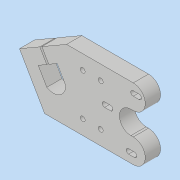
# Autodesk Inventor part: MMplate1
Saved by Autodesk Inventor 2017 (Build 210142000, 142)
## iProperties
Created: 2016-12-19
Part Number: MMplate1
Material: Generic
Document SubType Name: Modeling
Designer: Joshua Yuan
Density: 1 g/cm^3
Appearance: Default
Author: Joshua Yuan
Autodesk Inventor part; units mm, degrees
ref_plane "YZ Plane" through (0, 0, 0) normal (1, 0, 0) x (0, 1, 0)
ref_plane "XZ Plane" through (0, 0, 0) normal (0, 1, 0) x (-1, 0, 0)
ref_plane "XY Plane" through (0, 0, 0) normal (0, 0, 1) x (1, 0, 0)
sketch "sketch_plate" plane through (0, 0, 0) normal (0, 0, 1) x (1, 0, 0)
  line L0 (31.295, 48.2296) -> (38.3479, 52.3016)
  line L1 (47.1013, 57.4282) -> (54.2133, 45.1098)
  line L2 (31.295, 48.2296) -> (38.407, 35.9113)
  arc A0 (38.407, 35.9113) -> (54.2133, 45.1098) centre (43.8034, 44.8181) ccw
  line L3 (15.6813, 52.4133) -> (32.6329, 62.2003)
  line L4 (15.6813, 52.4133) -> (36.6325, 16.1248)
  line L5 (-9.4061, 0) -> (166.2056, 0) projected
  line L6 (0, -0.1502) -> (0, 91.4329) projected
  line L7 (34.3334, 63.2549) -> (40.0484, 53.3562)
  line L8 (32.6329, 62.2003) -> (38.3479, 52.3016)
  line L9 (34.3334, 63.2549) -> (54.8928, 75.1248)
  line L10 (40.0484, 53.3562) -> (47.1013, 57.4282)
  arc A1 (113.2079, 16.5197) -> (110.4273, 16.1948) centre (108.3973, 45.6248) ccw
  circle A2 centre (43.3573, 45.6248) radius 3.975 construction
  circle A3 centre (68.3573, 28.1248) radius 2.0193
  circle A4 centre (83.3573, 28.1248) radius 2.0193
  circle A5 centre (68.3573, 63.1248) radius 2.0193
  circle A6 centre (83.3573, 63.1248) radius 2.0193
  arc A7 (111.2231, 54.721) -> (117.8999, 44.9711) centre (108.3973, 45.6248) ccw
  circle A8 centre (86.5604, 47.5353) radius 2
  circle A9 centre (110.3078, 67.4617) radius 2
  circle A10 centre (130.2342, 43.7144) radius 2
  circle A11 centre (106.4868, 23.7879) radius 2
  line L11 (110.3078, 67.4617) -> (106.4868, 23.7879) construction
  line L12 (130.2342, 43.7144) -> (86.5604, 47.5353) construction
  circle A12 centre (91.5604, 47.5353) radius 2
  circle A13 centre (115.3078, 67.4617) radius 2
  circle A14 centre (111.4868, 23.7879) radius 2
  circle A15 centre (135.2342, 43.7144) radius 2
  circle A16 centre (110.4273, 45.6248) radius 29.5 construction
  circle A17 centre (110.4273, 45.6248) radius 9.525 construction
  line L13 (115.3078, 69.4617) -> (110.3078, 69.4617)
  line L14 (110.3078, 65.4617) -> (115.3078, 65.4617)
  line L15 (106.4868, 25.7879) -> (111.4868, 25.7879)
  line L16 (111.4868, 21.7879) -> (106.4868, 21.7879)
  line L17 (86.5604, 49.5353) -> (91.5604, 49.5353)
  line L18 (91.5604, 45.5353) -> (86.5604, 45.5353)
  line L19 (110.4273, 45.6248) -> (43.3573, 45.6248) construction
  circle A18 centre (88.5904, 47.5353) radius 2 construction
  circle A19 centre (112.3378, 67.4617) radius 2 construction
  circle A20 centre (132.2642, 43.7144) radius 2 construction
  circle A21 centre (108.5168, 23.7879) radius 2 construction
  line L20 (130.2342, 45.7144) -> (135.2342, 45.7144)
  line L21 (135.2342, 41.7144) -> (130.2342, 41.7144)
  line L22 (132.2642, 43.7144) -> (88.5904, 47.5353) construction
  line L23 (112.3378, 67.4617) -> (108.5168, 23.7879) construction
  line L24 (68.3573, 63.1248) -> (68.3573, 28.1248) construction
  line L25 (83.3573, 28.1248) -> (83.3573, 63.1248) construction
  arc A22 (110.4273, 55.1498) -> (110.4273, 75.1248) centre (110.4273, 65.1373) ccw
  arc A23 (110.4273, 16.1248) -> (110.4273, 36.0998) centre (110.4273, 26.1123) ccw
  line L26 (110.4273, 16.1248) -> (110.4273, 75.1248) construction
  line L27 (110.4273, 36.0998) -> (108.3973, 36.0998)
  line L28 (110.4273, 55.1498) -> (108.3973, 55.1498)
  arc A24 (117.8999, 44.9711) -> (111.2231, 54.721) centre (108.3973, 45.6248) ccw construction
  line L29 (108.3973, 16.1248) -> (36.6325, 16.1248)
  line L30 (54.8928, 75.1248) -> (110.4273, 75.1248)
  line L31 (110.4273, 16.1248) -> (108.3973, 16.1248)
  point P0 (114.7514, 74.4324)
  point P1 (112.8078, 65.4617)
  point P2 (108.3973, 45.6248)
  dimension "d8" = 18.288
  dimension "d9" = 14.224
  dimension "d10" = 10.414
  dimension "d13" = 11.43
  dimension "d14" = 11.43
  dimension "d15" = 2
  dimension "d17" = 59
  dimension "d18" = 7.95
  dimension "d19" = 9.144
  dimension "d20" = 9.2717
  dimension "d21" = 30
  dimension "d22" = 8.35
  dimension "d23" = 65.04
  dimension "d25" = 4.0386
  dimension "d26" = 4.0386
  dimension "d27" = 4.0386
  dimension "d28" = 4.0386
  dimension "d32" = 19.05
  dimension "d33" = 4
  dimension "d34" = 4
  dimension "d35" = 4
  dimension "d36" = 4
  dimension "d38" = 31
  dimension "d39" = 31
  dimension "d40" = 31
  dimension "d41" = 31
  dimension "d42" = 15
  dimension "d43" = 35
  dimension "d44" = 35
  dimension "d49" = 4
  dimension "d50" = 4
  dimension "d51" = 4
  dimension "d52" = 4
  dimension "d53" = 5
  dimension "d54" = 59
  dimension "d55" = 67.07
  dimension "d56" = 19.05
  dimension "d57" = 5
  dimension "d58" = 5
  dimension "d59" = 5
  dimension "d60" = 4
  dimension "d61" = 4
  dimension "d62" = 4
  dimension "d63" = 4
  dimension "d68" = 5
  dimension "d69" = 5
  dimension "d70" = 31
  dimension "d71" = 31
  dimension "d72" = 31
  dimension "d73" = 31
  dimension "d92" = 55.5345
  dimension "d95" = 25
  dimension "d87" = 4.0386
  constraints: 60 end point, 37 point on circle, 25 centre point, 18 tangent, 12 horizontal, 8 midpoint, 8 perpendicular, 7 point on line, 5 equal length, 5 parallel, 3 coincident, 3 vertical, 2 symmetric about line
  measures "d8" distance of L0.start L1.start
  measures "d9" distance of L0.start L2.end
  measures "d10" radius of A0
  measures "d13" distance between parallel lines of L4 L2
  measures "d14" distance of L7.start L7.end
  measures "d15" distance between parallel lines of L8 L7
  measures "d17" diameter of A1
  measures "d18" diameter of A2
  measures "d19" distance from line of L1 L19.end
  measures "d20" distance from line of L10 A0.centre
  measures "d21" angle of L5 L0
  measures "d22" distance from line of L10 L19.end
  measures "d23" distance of L19.end A1.centre
  measures "d25" diameter of A3
  measures "d26" diameter of A6
  measures "d27" diameter of A4
  measures "d28" diameter of A5
  measures "d32" diameter of A7
  measures "d33" diameter of A8
  measures "d34" diameter of A9
  measures "d35" diameter of A10
  measures "d36" diameter of A11
  measures "d38" distance of L12.start L11.end
  measures "d39" distance of L11.start L12.start
  measures "d40" distance of A8.centre L11.end
  measures "d41" distance of A8.centre L11.start
  measures "d42" distance of L24.start L25.end
  measures "d43" distance of L24.end L24.start
  measures "d44" distance of L25.start L25.end
  measures "d49" diameter of A12
  measures "d50" diameter of A13
  measures "d51" diameter of A14
  measures "d52" diameter of A15
  measures "d53" distance of A8.centre A12.centre
  measures "d54" diameter of A16
  measures "d55" distance of L19.end A16.centre
  measures "d56" diameter of A17
  measures "d57" distance of L11.end A14.centre
  measures "d58" distance of A15.centre L12.start
  measures "d59" distance of L11.start A13.centre
  measures "d60" diameter of A18
  measures "d61" diameter of A19
  measures "d62" diameter of A20
  measures "d63" diameter of A21
  measures "d68" angle of L19 L22
  measures "d69" angle of L19 L12
  measures "d70" distance of L22.start L23.start
  measures "d71" distance of L23.end L22.start
  measures "d72" distance of L23.end L22.end
  measures "d73" distance of L22.end L23.start
  measures "d92" distance of L9.end L26.end
  measures "d95" distance from line of L24 L19.end
extrude "Extrusion10" add sketch "sketch_plate" along normal blind 12.7 contours L2 A0 L1 L10 L7 L9 L30 A1 A6 A4 L29 L4 L3 L8 L0 | A1 A4 A6 A22 L28 A7 L27 A23 L31 | L30 A22 A1
body "Solid7"
body "Solid8"
